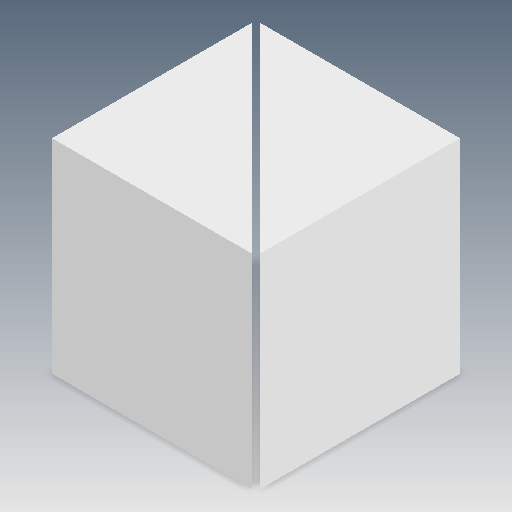
# Autodesk Inventor part: Beamsplittertransparent
Saved by Autodesk Inventor 2026 (Build 300175050, 175E)
## iProperties
Created: 2025-08-02
Part Number: Beamsplittertransparent
Material: Generic
Document SubType Name: Modeling
Designer: aman0
Density: 1 g/cm^3
Appearance: Default
Author: aman0
Autodesk Inventor part; units mm, degrees
ref_plane "YZ Plane" through (0, 0, 0) normal (1, 0, 0) x (0, 1, 0)
ref_plane "XZ Plane" through (0, 0, 0) normal (0, 1, 0) x (-1, 0, 0)
ref_plane "XY Plane" through (0, 0, 0) normal (0, 0, 1) x (1, 0, 0)
sketch "Sketch1" plane through (0, 0, 0) normal (0, 1, 0) x (-1, 0, 0)
  line L0 (-12.5, 12) -> (-12.5, -12.5)
  line L1 (-12.5, -12.5) -> (12, -12.5)
  line L2 (12.5, -12) -> (12.5, 12.5)
  line L3 (12.5, 12.5) -> (-12, 12.5)
  line L4 (-12.5, 12.5) -> (12.5, -12.5) construction
  line L5 (-12.5, -12.5) -> (12.5, 12.5) construction
  line L6 (12, -12.5) -> (-12.5, 12)
  line L7 (12.5, -12) -> (-12, 12.5)
  point P0 (0, 0)
  point P1 (0, 0)
  point P2 (0, 0)
  dimension "d0" = 25
  dimension "d1" = 25
  dimension "d2" = 0.5
  dimension "d3" = 0.5
  dimension "d4" = 0.5
  dimension "d5" = 0.7071
  dimension "d6" = 17.6777
  dimension "d7" = 17.6777
  dimension "d8" = 24.5
  constraints: 16 end point, 4 midpoint, 3 parallel, 1 perpendicular, 1 vertical
  measures "d0" distance of L4.start L0.end
  measures "d1" distance of L4.end L0.end
  measures "d2" distance of L1.end L4.end
  measures "d3" distance of L0.start L4.start
  measures "d4" distance of L3.end L4.start
  measures "d5" distance between parallel lines of L6 L7
  measures "d6" distance of point (0, 0) L2.end
  measures "d7" distance of point (0, 0) L0.end
  measures "d8" distance of L2.start L2.end
extrude "Extrusion1" add sketch "Sketch1" along normal mid plane 25
body "Solid1"
